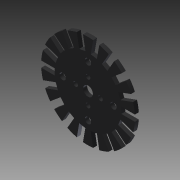
# Autodesk Inventor part: Plate 1
Saved by Autodesk Inventor 2015 (Build 190159000, 159)
## iProperties
Created: 2016-10-18
Part Number: Plate 1
Material: Generic
Document SubType Name: Modeling
Designer: James Yelland
Density: 1 g/cm^3
Appearance: Default
Author: James Yelland
Autodesk Inventor part; units mm, degrees
ref_plane "YZ Plane" through (0, 0, 0) normal (1, 0, 0) x (0, 1, 0)
ref_plane "XZ Plane" through (0, 0, 0) normal (0, 1, 0) x (-1, 0, 0)
ref_plane "XY Plane" through (0, 0, 0) normal (0, 0, 1) x (1, 0, 0)
sketch "Sketch1" plane through (0, 0, 0) normal (0, 1, 0) x (-1, 0, 0)
  circle A0 centre (0, 0) radius 24
  dimension "d0" = 48
  constraints: 1 centre point, 1 coincident
  measures "d0" diameter of A0
extrude "Extrusion1" add sketch "Sketch1" along normal blind 2
sketch "Sketch2" plane through (0, 2, 0) normal (0, 1, 0) x (1, 0, 0)
  circle A0 centre (0, 0) radius 24 projected
  line L0 (-24, 0) -> (-24, 1.6)
  line L1 (-24, 0) -> (-22.4, 0) construction
  line L2 (-24, 1.6) -> (-17, 1.6)
  line L3 (-17, 1.6) -> (-17, -1.6)
  line L4 (-17, -1.6) -> (-24, -1.6)
  line L5 (-24, -1.6) -> (-24, 1.6)
  line L6 (-22.5526, -8.2085) -> (-23.0999, -6.705)
  line L7 (-22.5526, -8.2085) -> (-21.0491, -7.6613) construction
  line L8 (-23.0999, -6.705) -> (-16.522, -4.3108)
  line L9 (-16.522, -4.3108) -> (-15.4275, -7.3179)
  line L10 (-15.4275, -7.3179) -> (-22.0054, -9.712)
  line L11 (-22.0054, -9.712) -> (-23.0999, -6.705)
  line L12 (-18.3851, -15.4269) -> (-19.4135, -14.2012)
  line L13 (-18.3851, -15.4269) -> (-17.1594, -14.3984) construction
  line L14 (-19.4135, -14.2012) -> (-14.0512, -9.7017)
  line L15 (-14.0512, -9.7017) -> (-11.9943, -12.1531)
  line L16 (-11.9943, -12.1531) -> (-17.3566, -16.6526)
  line L17 (-17.3566, -16.6526) -> (-19.4135, -14.2012)
  line L18 (-12, -20.7846) -> (-13.3856, -19.9846)
  line L19 (-12, -20.7846) -> (-11.2, -19.399) construction
  line L20 (-13.3856, -19.9846) -> (-9.8856, -13.9224)
  line L21 (-9.8856, -13.9224) -> (-7.1144, -15.5224)
  line L22 (-7.1144, -15.5224) -> (-10.6144, -21.5846)
  line L23 (-10.6144, -21.5846) -> (-13.3856, -19.9846)
  line L24 (-4.1676, -23.6354) -> (-5.7432, -23.3575)
  line L25 (-4.1676, -23.6354) -> (-3.8897, -22.0597) construction
  line L26 (-5.7432, -23.3575) -> (-4.5277, -16.4639)
  line L27 (-4.5277, -16.4639) -> (-1.3763, -17.0196)
  line L28 (-1.3763, -17.0196) -> (-2.5919, -23.9132)
  line L29 (-2.5919, -23.9132) -> (-5.7432, -23.3575)
  line L30 (4.1676, -23.6354) -> (2.5919, -23.9132)
  line L31 (4.1676, -23.6354) -> (3.8897, -22.0597) construction
  line L32 (2.5919, -23.9132) -> (1.3763, -17.0196)
  line L33 (1.3763, -17.0196) -> (4.5277, -16.4639)
  line L34 (4.5277, -16.4639) -> (5.7432, -23.3575)
  line L35 (5.7432, -23.3575) -> (2.5919, -23.9132)
  line L36 (12, -20.7846) -> (10.6144, -21.5846)
  line L37 (12, -20.7846) -> (11.2, -19.399) construction
  line L38 (10.6144, -21.5846) -> (7.1144, -15.5224)
  line L39 (7.1144, -15.5224) -> (9.8856, -13.9224)
  line L40 (9.8856, -13.9224) -> (13.3856, -19.9846)
  line L41 (13.3856, -19.9846) -> (10.6144, -21.5846)
  line L42 (18.3851, -15.4269) -> (17.3566, -16.6526)
  line L43 (18.3851, -15.4269) -> (17.1594, -14.3984) construction
  line L44 (17.3566, -16.6526) -> (11.9943, -12.1531)
  line L45 (11.9943, -12.1531) -> (14.0512, -9.7017)
  line L46 (14.0512, -9.7017) -> (19.4135, -14.2012)
  line L47 (19.4135, -14.2012) -> (17.3566, -16.6526)
  line L48 (22.5526, -8.2085) -> (22.0054, -9.712)
  line L49 (22.5526, -8.2085) -> (21.0491, -7.6613) construction
  line L50 (22.0054, -9.712) -> (15.4275, -7.3179)
  line L51 (15.4275, -7.3179) -> (16.522, -4.3108)
  line L52 (16.522, -4.3108) -> (23.0999, -6.705)
  line L53 (23.0999, -6.705) -> (22.0054, -9.712)
  line L54 (24, 0) -> (24, -1.6)
  line L55 (24, 0) -> (22.4, 0) construction
  line L56 (24, -1.6) -> (17, -1.6)
  line L57 (17, -1.6) -> (17, 1.6)
  line L58 (17, 1.6) -> (24, 1.6)
  line L59 (24, 1.6) -> (24, -1.6)
  line L60 (22.5526, 8.2085) -> (23.0999, 6.705)
  line L61 (22.5526, 8.2085) -> (21.0491, 7.6613) construction
  line L62 (23.0999, 6.705) -> (16.522, 4.3108)
  line L63 (16.522, 4.3108) -> (15.4275, 7.3179)
  line L64 (15.4275, 7.3179) -> (22.0054, 9.712)
  line L65 (22.0054, 9.712) -> (23.0999, 6.705)
  line L66 (18.3851, 15.4269) -> (19.4135, 14.2012)
  line L67 (18.3851, 15.4269) -> (17.1594, 14.3984) construction
  line L68 (19.4135, 14.2012) -> (14.0512, 9.7017)
  line L69 (14.0512, 9.7017) -> (11.9943, 12.1531)
  line L70 (11.9943, 12.1531) -> (17.3566, 16.6526)
  line L71 (17.3566, 16.6526) -> (19.4135, 14.2012)
  line L72 (12, 20.7846) -> (13.3856, 19.9846)
  line L73 (12, 20.7846) -> (11.2, 19.399) construction
  line L74 (13.3856, 19.9846) -> (9.8856, 13.9224)
  line L75 (9.8856, 13.9224) -> (7.1144, 15.5224)
  line L76 (7.1144, 15.5224) -> (10.6144, 21.5846)
  line L77 (10.6144, 21.5846) -> (13.3856, 19.9846)
  line L78 (4.1676, 23.6354) -> (5.7432, 23.3575)
  line L79 (4.1676, 23.6354) -> (3.8897, 22.0597) construction
  line L80 (5.7432, 23.3575) -> (4.5277, 16.4639)
  line L81 (4.5277, 16.4639) -> (1.3763, 17.0196)
  line L82 (1.3763, 17.0196) -> (2.5919, 23.9132)
  line L83 (2.5919, 23.9132) -> (5.7432, 23.3575)
  line L84 (-4.1676, 23.6354) -> (-2.5919, 23.9132)
  line L85 (-4.1676, 23.6354) -> (-3.8897, 22.0597) construction
  line L86 (-2.5919, 23.9132) -> (-1.3763, 17.0196)
  line L87 (-1.3763, 17.0196) -> (-4.5277, 16.4639)
  line L88 (-4.5277, 16.4639) -> (-5.7432, 23.3575)
  line L89 (-5.7432, 23.3575) -> (-2.5919, 23.9132)
  line L90 (-12, 20.7846) -> (-10.6144, 21.5846)
  line L91 (-12, 20.7846) -> (-11.2, 19.399) construction
  line L92 (-10.6144, 21.5846) -> (-7.1144, 15.5224)
  line L93 (-7.1144, 15.5224) -> (-9.8856, 13.9224)
  line L94 (-9.8856, 13.9224) -> (-13.3856, 19.9846)
  line L95 (-13.3856, 19.9846) -> (-10.6144, 21.5846)
  line L96 (-18.3851, 15.4269) -> (-17.3566, 16.6526)
  line L97 (-18.3851, 15.4269) -> (-17.1594, 14.3984) construction
  line L98 (-17.3566, 16.6526) -> (-11.9943, 12.1531)
  line L99 (-11.9943, 12.1531) -> (-14.0512, 9.7017)
  line L100 (-14.0512, 9.7017) -> (-19.4135, 14.2012)
  line L101 (-19.4135, 14.2012) -> (-17.3566, 16.6526)
  line L102 (-22.5526, 8.2085) -> (-22.0054, 9.712)
  line L103 (-22.5526, 8.2085) -> (-21.0491, 7.6613) construction
  line L104 (-22.0054, 9.712) -> (-15.4275, 7.3179)
  line L105 (-15.4275, 7.3179) -> (-16.522, 4.3108)
  line L106 (-16.522, 4.3108) -> (-23.0999, 6.705)
  line L107 (-23.0999, 6.705) -> (-22.0054, 9.712)
  point P0 (-17, 1.6)
  point P1 (-16.522, -4.3108)
  point P2 (-14.0512, -9.7017)
  point P3 (-11.9943, -12.1531)
  point P4 (-11.9943, -12.1531)
  point P5 (-9.8856, -13.9224)
  point P6 (-7.1144, -15.5224)
  point P7 (-7.1144, -15.5224)
  point P8 (-4.5277, -16.4639)
  point P9 (-1.3763, -17.0196)
  point P10 (-1.3763, -17.0196)
  point P11 (-4.5277, -16.4639)
  point P12 (1.3763, -17.0196)
  point P13 (4.5277, -16.4639)
  point P14 (1.3763, -17.0196)
  point P15 (7.1144, -15.5224)
  point P16 (9.8856, -13.9224)
  point P17 (9.8856, -13.9224)
  point P18 (7.1144, -15.5224)
  point P19 (11.9943, -12.1531)
  point P20 (14.0512, -9.7017)
  point P21 (14.0512, -9.7017)
  point P22 (15.4275, -7.3179)
  point P23 (16.522, -4.3108)
  point P24 (16.522, -4.3108)
  point P25 (15.4275, -7.3179)
  point P26 (17, -1.6)
  point P27 (17, 1.6)
  point P28 (17, 1.6)
  point P29 (16.522, 4.3108)
  point P30 (15.4275, 7.3179)
  point P31 (15.4275, 7.3179)
  point P32 (16.522, 4.3108)
  point P33 (14.0512, 9.7017)
  point P34 (11.9943, 12.1531)
  point P35 (11.9943, 12.1531)
  point P36 (14.0512, 9.7017)
  point P37 (9.8856, 13.9224)
  point P38 (7.1144, 15.5224)
  point P39 (7.1144, 15.5224)
  point P40 (9.8856, 13.9224)
  point P41 (4.5277, 16.4639)
  point P42 (1.3763, 17.0196)
  point P43 (1.3763, 17.0196)
  point P44 (4.5277, 16.4639)
  point P45 (-4.5277, 16.4639)
  point P46 (-4.5277, 16.4639)
  point P47 (-1.3763, 17.0196)
  point P48 (-7.1144, 15.5224)
  point P49 (-9.8856, 13.9224)
  point P50 (-9.8856, 13.9224)
  point P51 (-14.0512, 9.7017)
  point P52 (-16.522, 4.3108)
  point P53 (-16.522, 4.3108)
  dimension "d31" = 0
  dimension "d3" = 1.6
  dimension "d4" = 90
  dimension "d5" = 7
  dimension "d7" = 3.2
  dimension "d8" = 7
  dimension "d9" = 90
  dimension "d13" = 360
  constraints: 216 end point, 72 point on line, 4 vertical, 3 horizontal, 3 perpendicular, 2 coincident, 1 horizontal alignment, 522 other
  measures "d3" distance of L0.start L0.end
  measures "d4" angle of L1 L0
  measures "d5" distance of L0.end point (-17, 1.6)
  measures "d7" distance of point (-17, 1.6) point (-17, -1.6)
  measures "d8" distance of point (-17, -1.6) L4.end
  measures "d9" angle of L3 L4
extrude "Extrusion2" cut sketch "Sketch2" against normal blind 2 contours A0 L56 L57 L58 | L54 L56 A0 | A0 L58 L59 | L62 L63 L64 A0 | A0 L60 L62 | L52 L53 A0 | A0 L50 L51 L52 | A0 L64 L65 | L48 L50 A0 | L68 L69 L70 A0 | A0 L66 L68 | L46 L47 A0 | A0 L44 L45 L46 | A0 L70 L71 | L42 L44 A0 | L74 L75 L76 A0 | A0 L72 L74 | L40 L41 A0 | A0 L38 L39 L40 | A0 L76 L77 | L36 L38 A0 | L80 L81 L82 A0 | A0 L78 L80 | L34 L35 A0 | A0 L32 L33 L34 | A0 L82 L83 | L30 L32 A0 | L86 L87 L88 A0 | A0 L84 L86 | L28 L29 A0 | A0 L26 L27 L28 | A0 L88 L89 | L24 L26 A0 | L92 L93 L94 A0 | A0 L90 L92 | L22 L23 A0 | A0 L20 L21 L22 | A0 L94 L95 | L18 L20 A0 | L98 L99 L100 A0 | A0 L96 L98 | L16 L17 A0 | A0 L14 L15 L16 | A0 L100 L101 | L12 L14 A0 | L104 L105 L106 A0 | A0 L102 L104 | L10 L11 A0 | A0 L8 L9 L10 | A0 L106 L107 | L6 L8 A0 | L2 L3 L4 A0 | A0 L0 L2 | L4 L5 A0
sketch "Sketch3" plane through (0, 2, 0) normal (0, 1, 0) x (1, 0, 0)
  line L0 (0, 0) -> (-13, 0)
  circle A0 centre (-13, 0) radius 1.6
  circle A1 centre (0, -13) radius 1.6
  circle A2 centre (13, 0) radius 1.6
  circle A3 centre (0, 13) radius 1.6
  line L1 (0, 0) -> (6.35, 0)
  circle A4 centre (6.35, 0) radius 1.2
  circle A5 centre (0, 6.35) radius 1.2
  circle A6 centre (-6.35, 0) radius 1.2
  circle A7 centre (0, -6.35) radius 1.2
  circle A8 centre (0, 0) radius 2.5
  circle A9 centre (0, 0) radius 2.5
  dimension "d17" = 13
  dimension "d18" = 3.2
  dimension "d21" = 360
  dimension "d25" = 6.35
  dimension "d26" = 2.4
  dimension "d29" = 360
  dimension "d32" = 5
  dimension "d33" = 5
  constraints: 10 centre point, 4 coincident, 4 end point, 2 horizontal, 18 other
  measures "d17" distance of L0.start L0.end
  measures "d18" diameter of A0
  measures "d25" distance of L0.start L1.end
  measures "d26" diameter of A4
  measures "d32" diameter of A8
  measures "d33" diameter of A9
extrude "Extrusion3" cut sketch "Sketch3" against normal blind 2
body "Solid1"
